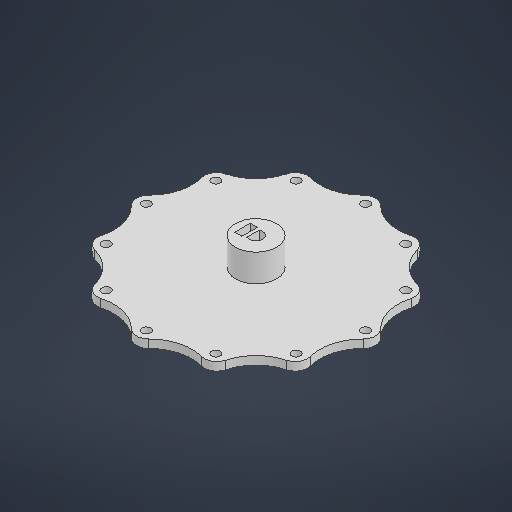
# Autodesk Inventor part: Shaft Collar
Saved by Autodesk Inventor 2025.1 (Build 291241000, 241)
## iProperties
Created: 2025-02-24
Part Number: Shaft Collar
Material: Generic
Document SubType Name: Modeling
Designer: jerem
Density: 1 g/cm^3
Appearance: Default
Author: jerem
Autodesk Inventor part; units mm, degrees
ref_plane "YZ Plane" through (0, 0, 0) normal (1, 0, 0) x (0, 1, 0)
ref_plane "XZ Plane" through (0, 0, 0) normal (0, 1, 0) x (-1, 0, 0)
ref_plane "XY Plane" through (0, 0, 0) normal (0, 0, 1) x (1, 0, 0)
sketch "Sketch1" plane through (0, 0, 0) normal (0, 1, 0) x (-1, 0, 0)
  circle A0 centre (0, 0) radius 2.5
  circle A1 centre (0, 0) radius 7.5
  circle A2 centre (0, 0) radius 39.5
  line L0 (1.0897, 2.25) -> (1.0897, -2.25)
  line L1 (1.0897, 0) -> (-2.5, 0) construction
  line L2 (-40, 0) -> (-40, 0) construction
  circle A3 centre (-40, 0) radius 1.6
  line L3 (0, 0) -> (-38.1541, 10.2234)
  line L4 (-38.1541, 10.2234) -> (-53.1259, 14.235) construction
  arc A4 (-42.2382, 3.2029) -> (-38.1541, 10.2234) centre (-53.1259, 14.235) ccw
  line L5 (-40, 0) -> (-43.5773, 0) construction
  arc A5 (-42.2382, 3.2029) -> (-43.5773, 0) centre (-39.0773, 0) ccw
  line L6 (0, 0) -> (-38.1541, -10.2234)
  arc A6 (-38.1541, -10.2234) -> (-42.2382, -3.2029) centre (-53.1259, -14.235) ccw
  arc A7 (-43.5773, 0) -> (-42.2382, -3.2029) centre (-39.0773, 0) ccw
  point P0 (-39.4711, 1.5101)
  point P1 (-39.4711, -1.5101)
  point P2 (-38.1541, -10.2234)
  point P3 (-38.1541, 10.2234)
  dimension "d0" = 5
  dimension "d1" = 4.5
  dimension "d2" = 5
  dimension "d3" = 15
  dimension "d4" = 79
  dimension "d21" = 3.2
  dimension "d23" = 40
  dimension "d45" = 15
  dimension "d46" = 31
  dimension "d48" = 39.5
  dimension "d49" = 4.5
  constraints: 14 end point, 11 point on circle, 8 centre point, 5 coincident, 3 symmetric about line, 2 horizontal, 2 line through centre, 1 collinear, 1 midpoint, 1 perpendicular, 1 tangent, 1 vertical, 2 other
  measures "d0" diameter of A0
  measures "d1" distance of L0.start L0.end
  measures "d2" radial gap between concentric circles of A0 A1
  measures "d3" diameter of A1
  measures "d4" diameter of A2
  measures "d21" diameter of A3
  measures "d23" distance of point (0, 0) L2.end
  measures "d45" angle of L1 L3
  measures "d46" diameter of A4
  measures "d48" distance of L3.end point (0, 0)
  measures "d49" radius of A5
extrude "Extrusion1" add sketch "Sketch1" along normal blind 3 contours A0 L0 | A0 L3 A1 L6 | A0 L6 A1 L3 | L3 A2 L6 A1 | A1 L6 A2 A3 L3 | A3 A2 picked at (-39.1312, 0)
extrude "Extrusion2" add sketch "Sketch1" along normal blind 10 from surface at 3 contours A0 L0 | A0 L3 A1 L6 | A0 L6 A1 L3
sketch "Sketch2" plane through (-1.0897, 0, 2.25) normal (1, 0, 0) x (0, 0, -1)
  line L0 (4.5, 13) -> (0, 13) projected
  line L1 (4.5, 13) -> (0, 13) projected
  line L2 (0, 0) -> (0, 13) projected
  line L3 (0, 0) -> (4.5, 0) projected
  line L4 (4.5, 0) -> (4.5, 13) projected
  circle A0 centre (2.25, 8) radius 1.6
  line L5 (2.25, 8) -> (2.25, 13) construction
  point P0 (2.25, 0)
  dimension "d9" = 3.2
  dimension "d10" = 5
  constraints: 2 end point, 1 centre point, 1 midpoint
  measures "d9" diameter of A0
  measures "d10" distance of L5.start L5.end
extrude "Extrusion3" cut sketch "Sketch2" against normal through all contours A0
sketch "Sketch3" plane through (0, 13, 0) normal (0, 1, 0) x (1, 0, 0)
  line L0 (-1.0897, 2.25) -> (-1.0897, -2.25) projected
  arc A0 (-1.0897, -2.25) -> (-1.0897, 2.25) centre (0, 0) ccw projected
  circle A1 centre (0, 0) radius 7.5 projected
  line L1 (-4.8897, -2.825) -> (-2.2897, -2.825)
  line L2 (-2.2897, -2.825) -> (-2.2897, 2.825)
  line L3 (-2.2897, 2.825) -> (-4.8897, 2.825)
  line L4 (-4.8897, 2.825) -> (-4.8897, -2.825)
  line L5 (-4.8897, -2.825) -> (-2.2897, 2.825) construction
  line L6 (-2.2897, -2.825) -> (-4.8897, 2.825) construction
  line L7 (-2.2897, 0) -> (-1.0897, 0) construction
  point P0 (-3.5897, 0)
  dimension "d13" = 1.2
  dimension "d14" = 5.65
  dimension "d15" = 2.6
  constraints: 14 end point, 4 midpoint, 2 parallel, 2 perpendicular, 1 horizontal
  measures "d13" distance of L7.start L7.end
  measures "d14" distance of L1.end L2.end
  measures "d15" distance of L2.end L3.end
ref_plane "Work Plane2" through (0, 8, 0) normal (0, 1, 0) x (1, 0, 0)
extrude "Extrusion4" cut sketch "Sketch3" along normal blind 10 and the other way blind 2.8 from surface at -5 contours L4 L3 L2 L1
extrude "Extrusion5" cut sketch "Sketch1" along normal through all contours A3 A2 picked at (-39.1312, 0)
extrude "Extrusion7" add sketch "Sketch1" along normal up to surface (3 mm away) contours A2 A3 A6 A7 A5 A4
pattern_circular "Circular Pattern1" count 12 over 360 about axis through (0, 0, 0) along (0, 1, 0) of "Extrusion5", "Extrusion7"
chamfer "Chamfer1" distance 1 angle 45 1 edges at (-1.0897, 0, 0)
equation "\"d48\" = 0.5 * d4"
body "Solid1"
